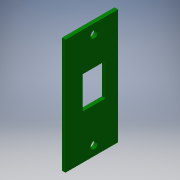
# Autodesk Inventor part: sensor_pcb
Saved by Autodesk Inventor 2018 (Build 220112000, 112)
## iProperties
Created: 2018-04-06
Part Number: sensor_pcb
Material: ガラス
Document SubType Name: Modeling
Designer: NaMACHAN
Density: 2.18 g/cm^3
Appearance: 濃いオリーブ
Author: NaMACHAN
Autodesk Inventor part; units mm, degrees
ref_plane "YZ Plane" through (0, 0, 0) normal (1, 0, 0) x (0, 1, 0)
ref_plane "XZ Plane" through (0, 0, 0) normal (0, 1, 0) x (-1, 0, 0)
ref_plane "XY Plane" through (0, 0, 0) normal (0, 0, 1) x (1, 0, 0)
sketch "スケッチ1" plane through (0, 0, 0) normal (1, 0, 0) x (0, 1, 0)
  line L0 (-11, -24) -> (11, -24)
  line L1 (11, -24) -> (11, 24)
  line L2 (11, 24) -> (-11, 24)
  line L3 (-11, 24) -> (-11, -24)
  line L4 (-11, -24) -> (11, 24) construction
  line L5 (11, -24) -> (-11, 24) construction
  point P0 (0, 0)
  dimension "d0" = 22
  dimension "d1" = 48
  constraints: 12 end point, 2 midpoint, 2 parallel, 1 horizontal, 1 perpendicular
  measures "d0" distance of L2.end L1.end
  measures "d1" distance of L1.end L0.end
extrude "押し出し1" add sketch "スケッチ1" along normal blind 1.5
sketch "スケッチ2" plane through (1.5, 0, 0) normal (1, 0, 0) x (0, 0, -1)
  line L0 (-24, 11) -> (-24, -11) projected
  line L1 (24, -11) -> (24, 11) projected
  line L2 (-24, -11) -> (24, -11) projected
  point P0 (0, 0)
  point P1 (-20, 1)
  point P2 (20, 1)
  dimension "d4" = 4
  dimension "d5" = 4
  dimension "d6" = 12
  constraints: 1 horizontal alignment
  measures "d4" distance from line of L0 point (-20, 1)
  measures "d5" distance from line of L1 point (20, 1)
  measures "d6" distance from line of L2 point (-20, 1)
hole "穴1" at (1.5, 1, 20) at (1.5, 1, -20) direction (-1, 0, 0) diameter 3 end through all
sketch "スケッチ3" plane through (0, 0, 0) normal (-1, 0, 0) x (0, 0, 1)
  line L0 (-5.5, -3.75) -> (8, -3.75)
  line L1 (8, -3.75) -> (8, 5.75)
  line L2 (8, 5.75) -> (-5.5, 5.75)
  line L3 (-5.5, 5.75) -> (-5.5, -3.75)
  line L4 (24, -11) -> (-24, -11) projected
  line L5 (-24, -11) -> (-24, 11) projected
  point P0 (0, 0)
  dimension "d14" = 7.25
  dimension "d15" = 18.5
  dimension "d16" = 32
  dimension "d17" = 16.75
  constraints: 8 end point, 2 parallel, 1 horizontal, 1 perpendicular
  measures "d14" distance between parallel lines of L4 L0
  measures "d15" distance between parallel lines of L5 L3
  measures "d16" distance between parallel lines of L5 L1
  measures "d17" distance between parallel lines of L4 L2
extrude "押し出し2" cut sketch "スケッチ3" against normal blind 1.5
